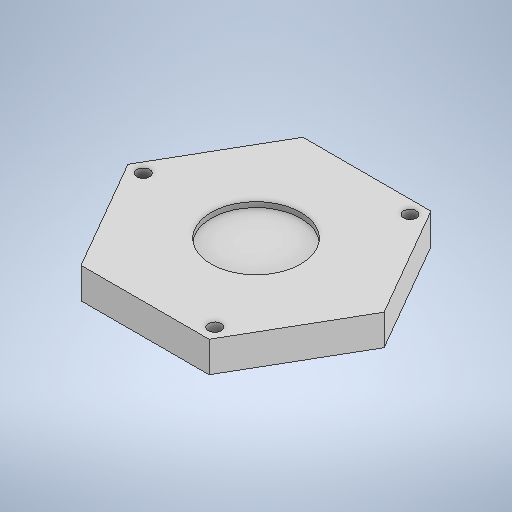
# Autodesk Inventor part: sensor 3
Saved by Autodesk Inventor 2025 (Build 290162000, 162)
## iProperties
Created: 2024-04-10
Part Number: sensor 3
Material: Generic
Document SubType Name: Modeling
Designer: mahal
Density: 1 g/cm^3
Appearance: Default
Author: mahal
Autodesk Inventor part; units mm, degrees
ref_plane "YZ Plane" through (0, 0, 0) normal (1, 0, 0) x (0, 1, 0)
sketch "Sketch1" plane through (0, 0, 0) normal (0, 1, 0) x (-1, 0, 0)
  line L0 (-25, -43.3013) -> (-50, 0)
  line L1 (-50, 0) -> (-25, 43.3013)
  line L2 (-25, 43.3013) -> (25, 43.3013)
  line L3 (25, 43.3013) -> (50, 0)
  line L4 (50, 0) -> (25, -43.3013)
  line L5 (25, -43.3013) -> (-25, -43.3013)
  point P0 (0, 0)
  point P1 (0, 0)
  dimension "d0" = 50
  constraints: 12 end point, 1 coincident, 13 other
  measures "d0" distance of L4.end L0.start
extrude "Extrusion1" add sketch "Sketch1" along normal blind 12
ref_plane "Work Plane1" through (0, 12, 0) normal (0, 1, 0) x (1, 0, 0)
sketch "Sketch2" plane through (0, 12, 0) normal (0, 1, 0) x (1, 0, 0)
  circle A0 centre (0, 0) radius 17.5
  dimension "d4" = 35
  constraints: 1 centre point, 1 coincident
  measures "d4" diameter of A0
extrude "Extrusion2" cut sketch "Sketch2" against normal blind 2
ref_plane "Work Plane2" through (0, 12, 0) normal (0, 1, 0) x (1, 0, 0)
sketch "Sketch3" plane through (0, 12, 0) normal (0, 1, 0) x (1, 0, 0)
  line L0 (-25, 43.3013) -> (-50, 0) projected
  line L1 (-50, 0) -> (-44, 0)
  circle A0 centre (-44, 0) radius 2.5
  line L2 (50, 0) -> (25, 43.3013) projected
  line L3 (25, 43.3013) -> (22, 38.1051)
  circle A1 centre (22, 38.1051) radius 2.5
  line L4 (25, -43.3013) -> (50, 0) projected
  line L5 (25, -43.3013) -> (22, -38.1051)
  circle A2 centre (22, -38.1051) radius 2.5
  point P0 (0, 0)
  dimension "d8" = 6
  dimension "d9" = 5
  dimension "d10" = 6
  dimension "d11" = 5
  dimension "d13" = 6
  dimension "d14" = 5
  constraints: 6 end point, 3 centre point, 3 coincident, 1 horizontal
  measures "d8" distance of L0.end L1.end
  measures "d9" diameter of A0
  measures "d10" distance of L2.end L3.end
  measures "d11" diameter of A1
  measures "d13" distance of L4.start L5.end
  measures "d14" diameter of A2
extrude "Extrusion3" cut sketch "Sketch3" against normal through all
body "Solid1"
